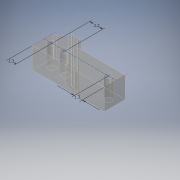
# Autodesk Inventor part: Bot_lateralized
Saved by Autodesk Inventor 2020 (Build 240168000, 168)
## iProperties
Created: 2019-02-01
Part Number: Bot_lateralized
Material: 일반
Document SubType Name: Modeling
Designer: Jeong Ji Hoon
Density: 1 g/cm^3
Appearance: 연회색 반사
Author: Jeong Ji Hoon
## iProperties of the stored document _3D 인쇄.ipt
Created: 2019-11-29
Part Number: _3D 인쇄
Material: 일반
Document SubType Name: Modeling
Designer: Knowblesse
Density: 1 g/cm^3
Appearance: 기본값
Author: Knowblesse
Autodesk Inventor part; units mm, degrees
ref_plane "YZ Plane" through (0, 0, 0) normal (1, 0, 0) x (0, 1, 0)
ref_plane "XZ Plane" through (0, 0, 0) normal (0, 1, 0) x (-1, 0, 0)
ref_plane "XY Plane" through (0, 0, 0) normal (0, 0, 1) x (1, 0, 0)
sketch "스케치1" plane through (0, 0, 0) normal (0, 1, 0) x (-1, 0, 0)
  line L0 (0, 0) -> (12, 0)
  line L1 (12, 0) -> (12, -4)
  line L2 (12, -4) -> (0, -4)
  line L3 (0, -4) -> (0, 0)
  dimension "d0" = 12
  dimension "d1" = 4
  constraints: 8 end point, 2 parallel, 1 horizontal, 1 perpendicular
  measures "d0" distance of L1.end L2.end
  measures "d1" distance of L0.end L1.end
extrude "돌출1" add sketch "스케치1" along normal blind 3.5
sketch "스케치2" plane through (0, 3.5, 0) normal (0, 1, 0) x (1, 0, 0)
  line L0 (0, 0) -> (0, 4) construction
  line L1 (0, 2) -> (-12, 2) construction
  line L2 (-12, 4) -> (-12, 0) construction
  point P0 (-1.3, 2)
  point P1 (-8.5, 2)
  point P2 (-10.7, 2)
  dimension "d59" = 1.3
  dimension "d60" = 2.2
  dimension "d62" = 1.3
  constraints: 3 point on line, 2 end point, 2 midpoint
  measures "d59" distance from line of L2 point (-10.7, 2)
  measures "d60" distance of point (-10.7, 2) point (-8.5, 2)
  measures "d62" distance from line of L0 point (-1.3, 2)
hole "구멍1" at (-10.7, 3.5, -2) at (-1.3, 3.5, -2) direction (0, -1, 0) diameter 1.1 end through all
hole "구멍2" at (-8.5, 3.5, -2) direction (0, -1, 0) diameter 1.2 end through all
sketch "스케치7" plane through (0, 0, -4) normal (0, 0, -1) x (-1, 0, 0)
  line L0 (12, 0) -> (0, 0) projected
  line L1 (12, 0) -> (12, 3.5) projected
  line L2 (0, 3.5) -> (12, 3.5) projected
  line L3 (0, 0) -> (0, 3.5) projected
  point P0 (0, 0)
extrude "돌출5" cut sketch "스케치7" against normal blind 0.5
sketch "스케치8" plane through (0, 0, -3.5) normal (0, 0, -1) x (-1, 0, 0)
  line L0 (0, 0) -> (0, 3.5) projected
  line L1 (12, 0) -> (0, 0) projected
  line L2 (12, 3.5) -> (12, 0) projected
  line L3 (0, 3.5) -> (12, 3.5) projected
  line L4 (12, 3.5) -> (0, 3.5) projected
  line L5 (10.5, 3.5) -> (8.9, 3.5)
  line L6 (8.9, 3.5) -> (8.9, -4)
  line L7 (8.9, -4) -> (10.5, -4)
  line L8 (10.5, -4) -> (10.5, 3.5)
  point P0 (0, 0)
  point P1 (10.5, 3.5)
  dimension "d78" = 1.5
  dimension "d79" = 1.6
  dimension "d92" = 4
  constraints: 8 end point, 2 parallel, 1 horizontal, 1 perpendicular, 1 point on line
  measures "d78" distance between parallel lines of L2 L8
  measures "d79" distance between parallel lines of L8 L6
  measures "d92" distance between parallel lines of L1 L7
extrude "돌출6" add sketch "스케치8" along normal blind 1.5 contours L6 L3 L8 L1 | L1 L8 L7 L6
chamfer "모따기1" distance 1 angle 45 2 edges at (-8.9, 1.75, -3.5) (-10.5, 1.75, -3.5)
chamfer "모따기2" distance 0.5 angle 45 2 edges at (-10.5, 0, -4) (-8.9, 0, -4)
sketch "스케치9" plane through (0, 0, -5) normal (0, 0, -1) x (-1, 0, 0)
  line L0 (10.5, 3.5) -> (8.9, 3.5) projected
  line L1 (8.9, 3.5) -> (8.9, -4) projected
  line L2 (8.9, -4) -> (10.5, -4) projected
  line L3 (10.5, -4) -> (10.5, 3.5) projected
  line L4 (8.9, -4) -> (10.5, -4) projected
  line L5 (0, 0) -> (12, 0) projected
  line L6 (9.2, -4) -> (10.2, -4)
  line L7 (10.2, -4) -> (10.2, 0)
  line L8 (10.2, 0) -> (9.2, 0)
  line L9 (9.2, 0) -> (9.2, -4)
  line L10 (9.2, 0) -> (10.2, 0)
  line L11 (10.2, 0) -> (10.2, 3.5)
  line L12 (10.2, 3.5) -> (9.2, 3.5)
  line L13 (9.2, 3.5) -> (9.2, 0)
  line L14 (10.5, 3.5) -> (8.9, 3.5) projected
  point P0 (9.7, -4)
  point P1 (9.2, 0)
  point P2 (9.2, 0)
  point P3 (10.2, 0)
  dimension "d83" = 1
  constraints: 16 end point, 4 parallel, 2 collinear, 2 horizontal, 2 midpoint, 2 perpendicular, 2 point on line
  measures "d83" distance between parallel lines of L9 L7
extrude "돌출7" cut sketch "스케치9" against normal blind 0.2 contours L11 L5 L13 L0 | L7 L2 L9 L5
sketch "스케치10" plane through (0, 0, -3.5) normal (0, 0, 1) x (1, 0, 0)
  line L0 (-8.9, -0.5) -> (-8.9, -4) projected
  line L1 (-8.4, 0) -> (-8.9, -0.5) projected
  line L2 (-11, 0) -> (-8.4, 0) projected
  line L3 (-10.5, -0.5) -> (-11, 0) projected
  line L4 (-10.5, -4) -> (-10.5, -0.5) projected
  line L5 (-8.9, -4) -> (-10.5, -4) projected
  point P0 (0, 0)
extrude "돌출8" cut sketch "스케치10" against normal blind 0.5
chamfer "모따기5" distance 0.5 distance2 1 1 edges at (-9.7, -4, -4) measured on face at (-9.7, -4, -4.5)
equation "\"G23_F\" = 0.65"
equation "\"G23_M\" = 0.67"
equation "\"Screw_F\" = 1.3"
equation "\"Screw_M\" = 1.6"
